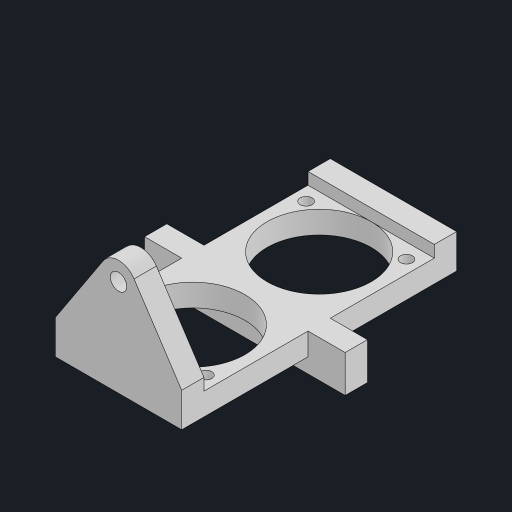
# Autodesk Inventor part: Ultrasonic_holderV3
Saved by Autodesk Inventor 2023 (Build 270158000, 158)
## iProperties
Created: 2022-06-24
Part Number: Ultrasonic_holderV3
Material: 一般
Document SubType Name: Modeling
Designer: legot
Density: 1 g/cm^3
Appearance: 既定
Author: legot
Autodesk Inventor part; units mm, degrees
ref_plane "YZ Plane" through (0, 0, 0) normal (1, 0, 0) x (0, 1, 0)
ref_plane "XZ Plane" through (0, 0, 0) normal (0, 1, 0) x (-1, 0, 0)
ref_plane "XY Plane" through (0, 0, 0) normal (0, 0, 1) x (1, 0, 0)
sketch "スケッチ1" plane through (0, 0, 0) normal (0, 1, 0) x (-1, 0, 0)
  line L0 (8.5, 15.5) -> (-8.5, 15.5) construction
  line L1 (-8.5, 15.5) -> (-8.5, -15.5)
  line L2 (-8.5, -15.5) -> (8.5, -15.5) construction
  line L3 (8.5, -15.5) -> (8.5, 15.5)
  circle A0 centre (0, 8.5) radius 7
  circle A1 centre (0, -8.5) radius 7
  circle A2 centre (6.75, -13.5) radius 0.8
  line L4 (6.75, -13.5) -> (-6.75, -13.5) construction
  line L5 (-6.75, -13.5) -> (-6.75, 13.5) construction
  line L6 (-6.75, 13.5) -> (6.75, 13.5) construction
  line L7 (6.75, 13.5) -> (6.75, -13.5) construction
  circle A3 centre (-6.75, -13.5) radius 0.8
  circle A4 centre (6.75, 13.5) radius 0.8
  circle A5 centre (-6.75, 13.5) radius 0.8
  line L8 (8.5, 18.5) -> (-8.5, 18.5)
  line L9 (-8.5, 18.5) -> (-8.5, 15.5)
  line L10 (-8.5, 15.5) -> (8.5, 15.5)
  line L11 (8.5, 15.5) -> (8.5, 18.5)
  line L12 (8.5, -15.5) -> (-8.5, -15.5)
  line L13 (-8.5, -15.5) -> (-8.5, -18.5)
  line L14 (-8.5, -18.5) -> (8.5, -18.5)
  line L15 (8.5, -18.5) -> (8.5, -15.5)
  line L16 (-6.75, 10.354) -> (-6.75, -10.354)
  line L17 (13.5, -1.5) -> (-13.5, -1.5)
  line L18 (-13.5, -1.5) -> (-13.5, 1.5)
  line L19 (-13.5, 1.5) -> (13.5, 1.5)
  line L20 (13.5, 1.5) -> (13.5, -1.5)
  point P0 (0, 0)
  point P1 (0, 0)
  point P2 (0, 15.5)
  point P3 (8.5, 0)
  point P4 (6.75, 0)
  point P5 (0, 13.5)
  point P6 (6.75, 10.354)
  point P7 (6.75, -10.354)
  point P8 (7, 8.5)
  point P9 (7, -8.5)
  point P10 (-7, 8.5)
  point P11 (-7, -8.5)
  point P12 (-6.75, -6.646)
  point P13 (-6.75, 6.646)
  point P14 (13.5, 0)
  point P15 (0, -1.5)
  point P16 (8.5, 1.5)
  point P17 (8.5, -1.5)
  point P18 (-8.5, -1.5)
  point P19 (-8.5, 1.5)
  dimension "d0" = 17
  dimension "d1" = 31
  dimension "d2" = 14
  dimension "d4" = 27
  dimension "d5" = 13.5
  dimension "d7" = 1.6
  dimension "d9" = 3
  dimension "d26" = 5
  constraints: 42 end point, 10 parallel, 8 point on circle, 6 centre point, 6 midpoint, 6 point on line, 5 coincident, 5 horizontal, 5 perpendicular, 5 vertical alignment, 4 equal radius, 3 horizontal alignment, 3 tangent, 1 collinear
  measures "d0" distance of L3.end L1.start
  measures "d1" distance of L3.start L3.end
  measures "d2" diameter of A0
  measures "d4" distance of L7.start L7.end
  measures "d5" distance of L7.end L5.start
  measures "d7" diameter of A4
  measures "d9" distance of L10.end L8.start
  measures "d26" distance between parallel lines of L1 L18
extrude "押し出し1" add sketch "スケッチ1" against normal blind 3 contours L10 A0 L16 L19 L1 | L9 L8 L11 L10 | L19 L16 L17 L1 | L1 L17 L18 L19 | L10 L3 L19 A0 | L17 L16 A1 L12 L1 | L19 L3 L17 L16 | L16 A0 L19 | L12 L15 L14 L13 | L17 A1 L16 | L19 L20 L17 L3 | A1 L17 L3 L12
extrude "押し出し2" add sketch "スケッチ1" along normal blind 1.6 contours L9 L8 L11 L10 | L12 L15 L14 L13
sketch "スケッチ4" plane through (0, -3, 0) normal (0, -1, 0) x (1, 0, 0)
  line L0 (-8.5, 1.5) -> (-13.5, 1.5) projected
  line L1 (-13.5, 1.5) -> (-13.5, -1.5) projected
  line L2 (-13.5, -1.5) -> (-8.5, -1.5) projected
  line L3 (8.5, -1.5) -> (13.5, -1.5) projected
  line L4 (13.5, -1.5) -> (13.5, 1.5) projected
  line L5 (13.5, 1.5) -> (8.5, 1.5) projected
  line L6 (-13.5, -1.5) -> (13.5, -1.5) projected
  line L7 (-8.5, 1.5) -> (-13.5, 1.5) projected
  line L8 (-13.5, 1.5) -> (13.5, 1.5)
  line L9 (13.5, 1.5) -> (13.5, -1.5)
  line L10 (13.5, -1.5) -> (-13.5, -1.5)
  line L11 (-13.5, -1.5) -> (-13.5, 1.5)
  point P0 (-7, -1.5)
  point P1 (7, -1.5)
  point P2 (7, 1.5)
  point P3 (-7, 1.5)
  point P4 (0, 0)
  point P5 (-8.5, -1.5)
  point P6 (7, -1.5)
  point P7 (8.5, -1.5)
  point P8 (8.5, 1.5)
  point P9 (-7, 1.5)
  constraints: 8 end point, 2 parallel, 1 horizontal, 1 perpendicular
extrude "押し出し4" add sketch "スケッチ4" along normal blind 2
sketch "スケッチ2" plane through (-8.5, -3, 18.5) normal (0, 0, 1) x (1, 0, 0)
  line L0 (0, 4.6) -> (17, 4.6) projected
  circle A0 centre (8.5, 13) radius 2.5
  line L1 (17, 4.6) -> (0, 4.6) projected
  line L2 (0, 4.6) -> (6.4096, 14.3712)
  line L3 (17, 4.6) -> (10.5904, 14.3712)
  point P0 (8.5, 3)
  dimension "d14" = 10
  dimension "d15" = 5
  constraints: 4 end point, 2 point on circle, 2 tangent, 1 centre point, 1 vertical alignment
  measures "d14" distance of A0.centre point (8.5, 3)
  measures "d15" diameter of A0
extrude "押し出し3" add sketch "スケッチ2" against normal up to surface (3 mm away)
sketch "スケッチ3" plane through (-8.5, -3, 18.5) normal (0, 0, 1) x (1, 0, 0)
  arc A0 (10.5904, 14.3712) -> (6.4096, 14.3712) centre (8.5, 13) ccw projected
  point P0 (8.5, 3)
  constraints: 1 coincident
hole "穴1" at (0, 10, 18.5) direction (0, 0, -1) diameter 2.2 end through all
